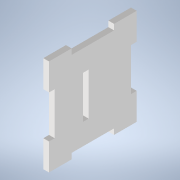
# Autodesk Inventor part: Platte2-Seite
Saved by Autodesk Inventor 2020.3 (Build 243373010, 373A)
## iProperties
Created: 2020-11-28
Part Number: Platte2-Seite
Material: Generisch
Document SubType Name: Modeling
Designer: Stefan
Density: 1 g/cm^3
Appearance: Vorgabe
Author: Stefan
Autodesk Inventor part; units mm, degrees
ref_plane "YZ Plane" through (0, 0, 0) normal (1, 0, 0) x (0, 1, 0)
ref_plane "XZ Plane" through (0, 0, 0) normal (0, 1, 0) x (-1, 0, 0)
ref_plane "XY Plane" through (0, 0, 0) normal (0, 0, 1) x (1, 0, 0)
sketch "Skizze1" plane through (0, 0, 0) normal (1, 0, 0) x (0, 1, 0)
  line L0 (5.6933, -1.6012) -> (5.6933, -11.6012)
  line L1 (5.6933, -11.6012) -> (-69.3067, -11.6012)
  line L2 (-69.3067, -11.6012) -> (-69.3067, -1.6012)
  line L3 (-116.8067, -1.6012) -> (-69.3067, -1.6012)
  line L4 (5.6933, -1.6012) -> (53.1933, -1.6012)
  line L5 (5.6933, -156.6012) -> (5.6933, -146.6012)
  line L6 (5.6933, -146.6012) -> (-69.3067, -146.6012)
  line L7 (-69.3067, -146.6012) -> (-69.3067, -156.6012)
  line L8 (-69.3067, -61.6012) -> (5.6933, -61.6012)
  line L9 (5.6933, -61.6012) -> (5.6933, -71.6012)
  line L10 (5.6933, -71.6012) -> (-69.3067, -71.6012)
  line L11 (-69.3067, -71.6012) -> (-69.3067, -61.6012)
  line L12 (53.1933, -156.6012) -> (5.6933, -156.6012)
  line L13 (-69.3067, -156.6012) -> (-116.8067, -156.6012)
  line L14 (-116.8067, -41.6012) -> (-106.8067, -41.6012)
  line L15 (-106.8067, -41.6012) -> (-106.8067, -116.6012)
  line L16 (-106.8067, -116.6012) -> (-116.8067, -116.6012)
  line L17 (-116.8067, -156.6012) -> (-116.8067, -116.6012)
  line L18 (-116.8067, -41.6012) -> (-116.8067, -1.6012)
  line L19 (53.1933, -41.6012) -> (43.1933, -41.6012)
  line L20 (43.1933, -41.6012) -> (43.1933, -116.6012)
  line L21 (43.1933, -116.6012) -> (53.1933, -116.6012)
  line L22 (53.1933, -1.6012) -> (53.1933, -41.6012)
  line L23 (53.1933, -116.6012) -> (53.1933, -156.6012)
  point P0 (0, 0)
  dimension "d0" = 170
  dimension "d1" = 155
  dimension "d2" = 75
  dimension "d3" = 10
  dimension "d5" = 75
  dimension "d6" = 10
  dimension "d8" = 75
  dimension "d9" = 10
  dimension "d10" = 50
  dimension "d14" = 0
  dimension "d15" = 0
  dimension "d16" = 10
  dimension "d17" = 75
  dimension "d18" = 40
  dimension "d19" = 0
  dimension "d20" = 10
  dimension "d23" = 40
  dimension "d24" = 10
  dimension "d25" = 47.5
  dimension "d26" = 37.5
  dimension "d27" = 40
  dimension "d28" = 75
  dimension "d29" = 170
  constraints: 48 end point, 14 parallel, 7 perpendicular, 5 horizontal
  measures "d0" distance of L3.start L4.end
  measures "d1" distance of L4.end L12.start
  measures "d2" distance of L0.end L1.end
  measures "d3" distance of L0.start L0.end
  measures "d5" distance of L6.end L5.end
  measures "d6" distance of L5.end L5.start
  measures "d8" distance of L9.end L10.end
  measures "d9" distance of L8.end L9.end
  measures "d10" distance between parallel lines of L8 L1
  measures "d14" distance between parallel lines of L11 L7
  measures "d15" distance between parallel lines of L2 L11
  measures "d16" distance of L15.end L16.end
  measures "d17" distance of L14.end L15.end
  measures "d18" distance between parallel lines of L14 L3
  measures "d19" distance between parallel lines of L4 L3
  measures "d20" distance of L21.end L20.end
  measures "d23" distance between parallel lines of L16 L13
  measures "d24" distance of L6.end L7.end
  measures "d25" distance of L3.start L2.end
  measures "d26" distance between parallel lines of L9 L20
  measures "d27" distance of L4.end L19.start
  measures "d28" distance of L19.end L20.end
  measures "d29" distance between parallel lines of L23 L17
extrude "Extrusion1" add sketch "Skizze1" along normal blind 10
